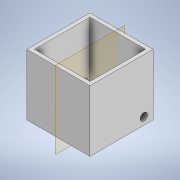
# Autodesk Inventor part: waterBallonHolderv1
Saved by Autodesk Inventor 2020 (Build 240168000, 168)
## iProperties
Created: 2022-09-14
Part Number: waterBallonHolderv1
Material: Generic
Document SubType Name: Sheet Metal
Designer: kouda
Density: 1 g/cm^3
Appearance: Default
Sheet Metal Rule: Default
Author: kouda
Autodesk Inventor part; units mm, degrees
ref_plane "YZ Plane" through (0, 0, 0) normal (1, 0, 0) x (0, 1, 0)
ref_plane "XZ Plane" through (0, 0, 0) normal (0, 1, 0) x (-1, 0, 0)
ref_plane "XY Plane" through (0, 0, 0) normal (0, 0, 1) x (1, 0, 0)
sketch "Sketch1" plane through (0, 0, 0) normal (0, 1, 0) x (-1, 0, 0)
  line L0 (0, 0) -> (-34, 0)
  line L1 (-34, 0) -> (-34, 34)
  line L2 (-34, 34) -> (0, 34)
  line L3 (0, 34) -> (0, 0)
  dimension "d0" = 34
  dimension "d1" = 34
  constraints: 8 end point, 2 parallel, 1 horizontal, 1 perpendicular
  measures "d0" distance of L1.end L2.end
  measures "d1" distance of L0.end L1.end
extrude "Extrusion1" add sketch "Sketch1" along normal blind 33
sketch "Sketch2" plane through (0, 33, 0) normal (0, 1, 0) x (1, 0, 0)
  line L0 (0, -34) -> (34, -34) projected
  line L1 (34, -34) -> (34, 0) projected
  line L2 (34, 0) -> (0, 0) projected
  line L3 (0, 0) -> (0, -34) projected
  line L4 (2, -2) -> (32, -2)
  line L5 (32, -2) -> (32, -32)
  line L6 (32, -32) -> (2, -32)
  line L7 (2, -32) -> (2, -2)
  dimension "d4" = 2
  constraints: 8 end point, 3 other
  measures "d4" distance between parallel lines of L2 L4
extrude "Extrusion2" cut sketch "Sketch2" against normal blind 36 contours L4 L5 L6 L7
sketch "Sketch3" plane through (34, 0, 34) normal (1, 0, 0) x (0, 0, -1)
  line L0 (0, 0) -> (34, 0) projected
  line L1 (0, 33) -> (34, 33) projected
  line L2 (2, 33) -> (32, 33) projected
  line L3 (34, 0) -> (34, 38) projected
  line L4 (34, 0) -> (29, 0)
  line L5 (0, 0) -> (34, 0) projected
  line L6 (29, 0) -> (29, 4)
  line L7 (34, 0) -> (34, 33) projected
  line L8 (0, 0) -> (0, 33) projected
  line L9 (32, 0) -> (2, 0) projected
  line L10 (32, 33) -> (32, 0) projected
  line L11 (2, 33) -> (2, 0) projected
  dimension "d7" = 5
  dimension "d8" = 4
  constraints: 4 end point, 1 coincident, 1 perpendicular, 1 point on line
  measures "d7" distance of L3.start L4.end
  measures "d8" distance of L4.end L6.end
hole "Hole1" at (34, 4, 5) direction (-1, 0, 0) diameter 4 depth 2
ref_plane "Work Plane1" through (17, 33, 32) normal (1, 0, 0) x (0, 0, -1)
mirror "Mirror1" about plane through (17, 33, 32) normal (1, 0, 0) of "Hole1"
sketch "Sketch6" plane through (0, 33, 0) normal (0, 1, 0) x (1, 0, 0)
  point P0 (0, 0)
sketch "Sketch7" plane through (0, 0, 0) normal (0, -1, 0) x (1, 0, 0)
  line L0 (34, 0) -> (0, 0) projected
  line L1 (0, 34) -> (34, 34) projected
  line L2 (34, 0) -> (0, 0)
  line L3 (0, 0) -> (0, 34)
  line L4 (0, 34) -> (34, 34)
  line L5 (34, 34) -> (34, 0)
  constraints: 8 end point, 2 parallel, 1 horizontal, 1 perpendicular
extrude "Extrusion5" add sketch "Sketch7" against normal blind 2
equation "\"BendRadius\" = Thickness"
equation "\"BendReliefWidth\" = Thickness"
equation "\"BendReliefDepth\" = 0.5 * Thickness"
equation "\"CornerReliefSize\" = 4 * Thickness"
equation "\"MinimumRemnant\" = 2 * Thickness"
equation "\"TransitionRadius\" = BendRadius"
equation "\"JacobiRadiusSize\" = Thickness"
equation "\"GapSize\" = Thickness"
equation "\"Thickness\" = 0.5"
body "Solid1"
